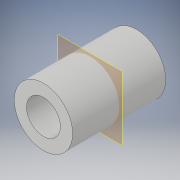
# Autodesk Inventor part: Machinable Bore Flexible Shaft Coupling
Saved by Autodesk Inventor 2018 (Build 220112000, 112)
## iProperties
Created: 2020-03-23
Part Number: Machinable Bore Flexible Shaft Coupling
Material: Generic
Document SubType Name: Modeling
Designer: emile
Density: 1 g/cm^3
Appearance: Default
Catalog Web Link: https://www.mcmaster.com/3530n111
Author: emile
Autodesk Inventor part; units mm, degrees
ref_plane "YZ Plane" through (0, 0, 0) normal (1, 0, 0) x (0, 1, 0)
ref_plane "XZ Plane" through (0, 0, 0) normal (0, 1, 0) x (-1, 0, 0)
ref_plane "XY Plane" through (0, 0, 0) normal (0, 0, 1) x (1, 0, 0)
sketch "Sketch1" plane through (0, 0, 0) normal (0, 0, 1) x (1, 0, 0)
  circle A0 centre (0, 0) radius 7.9375
  circle A1 centre (0, 0) radius 13.6922
  dimension "d0" = 15.875
  dimension "d1" = 27.3844
  constraints: 2 centre point, 2 coincident
  measures "d0" diameter of A0
  measures "d1" diameter of A1
extrude "Extrusion1" add sketch "Sketch1" along normal blind 43.6562
ref_plane "Work Plane1" through (0, 0, 21.8281) normal (0, 0, 1) x (1, 0, 0)
sketch "Sketch3" plane through (0, 0, 21.8281) normal (0, 0, 1) x (1, 0, 0)
  circle A0 centre (0, 0) radius 7.9375 projected
extrude "Extrusion2" add sketch "Sketch3" along normal mid plane 12.7
sketch "Sketch5" plane through (0, 0, 0) normal (0, 0, -1) x (-1, 0, 0)
  circle A0 centre (0, 0) radius 3.175
  circle A1 centre (0, 0) radius 13.6922 projected
  circle A2 centre (0, 0) radius 7.9375 projected
  dimension "d6" = 6.35
  constraints: 1 centre point, 1 coincident
  measures "d6" diameter of A0
extrude "Extrusion3" add sketch "Sketch5" against normal up to surface (15.4781 mm away) contours A2
body "Solid1"
